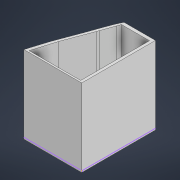
# Autodesk Inventor part: phoneBucketV2
Saved by Autodesk Inventor 2022 (Build 260153000, 153)
## iProperties
Created: 2022-07-18
Part Number: phoneBucketV2
Material: Generic
Document SubType Name: Modeling
Designer: matti
Density: 1 g/cm^3
Appearance: Default
Author: matti
Autodesk Inventor part; units mm, degrees
ref_plane "YZ Plane" through (0, 0, 0) normal (1, 0, 0) x (0, 1, 0)
ref_plane "XZ Plane" through (0, 0, 0) normal (0, 1, 0) x (-1, 0, 0)
ref_plane "XY Plane" through (0, 0, 0) normal (0, 0, 1) x (1, 0, 0)
sketch "Sketch1" plane through (0, 0, 0) normal (0, 1, 0) x (-1, 0, 0)
  line L0 (4, -2.4997) -> (79.711, -2.4997)
  line L1 (4, -103.4997) -> (4, -2.4997)
  line L2 (45, -103.4997) -> (4, -103.4997)
  line L3 (69.7122, -36.1325) -> (54.8327, -76.055)
  line L4 (54.8327, -76.055) -> (53.637, -79.4997)
  line L5 (53.637, -79.4997) -> (47.0364, -98.0359)
  line L6 (47.0364, -98.0359) -> (45, -103.4997)
  line L7 (79.711, -2.4997) -> (69.7122, -36.1325)
  line L8 (84.9819, 0) -> (0, 0)
  line L9 (75.6001, -30.2846) -> (84.9819, 0)
  line L10 (84.9819, 0) -> (75.6001, -30.2846)
  line L11 (70.9666, -42.7177) -> (65.5988, -57.1214)
  line L12 (61.2006, -68.9229) -> (56.067, -83.7178)
  line L13 (75.6001, -30.2846) -> (61.2006, -68.9229)
  line L14 (47.8016, -104.8767) -> (46.0595, -108.2232)
  line L15 (50.5948, -98.4014) -> (47.8016, -104.8767)
  line L16 (56.067, -83.7178) -> (50.5948, -98.4014)
  line L17 (0, -108.2232) -> (0, 0)
  line L18 (46.0595, -108.2232) -> (0, -108.2232)
  point P0 (0, 0)
  point P1 (-1, 0)
  constraints: 38 end point, 2 perpendicular
extrude "Extrusion1" add sketch "Sketch1" against normal blind 2.5 contours L0 L7 L3 L4 L5 L6 L2 L1 | L9 L13 L11 L12 L16 L15 L14 L18 L17 L8
extrude "Extrusion2" add sketch "Sketch1" along normal blind 111.5
body "Solid1"
